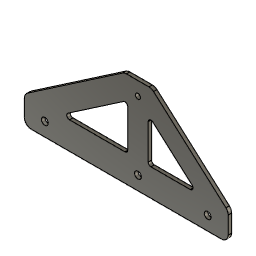
New Bell Crank with Variables v8 (Autodesk Fusion 360 design; units mm, degrees)
Autodesk Fusion 360 part; units mm, degrees
note: some values were not read from the file. Set by a fixed rule: which sketch regions a step uses.
sketch "Base Bell Crank" plane through (0, 0, 0) normal (0, 1, 0) x (1, 0, 0)
  circle A0 centre (64.9712, 0) radius 3.175
  circle A1 centre (-86.6283, 0) radius 3.175
  circle A2 centre (0, -63.5) radius 2.3813
  circle A3 centre (0, 0) radius 3.175
  line L0 (0, -63.5) -> (0, 0) construction
  line L1 (0, 0) -> (64.9712, 0) construction
  line L2 (0, 0) -> (-86.6283, 0) construction
  line L3 (-12.7, -76.2) -> (12.7, -76.2)
  line L4 (12.7, -76.2) -> (84.0212, -12.7)
  line L5 (-105.6783, 12.7) -> (-105.6783, -12.7)
  line L6 (0, -63.5) -> (0, -76.2) construction
  line L7 (64.9712, 0) -> (84.0212, 0) construction
  line L8 (84.0212, -12.7) -> (84.0212, 12.7)
  line L9 (-105.6783, 12.7) -> (84.0212, 12.7)
  line L10 (-105.6783, -12.7) -> (-12.7, -76.2)
  dimension "d12" = 4.7625
  dimension "d13" = 6.35
  dimension "d19" = 6.35
  dimension "d20" = 63.5
  dimension "d21" = 64.9712
  dimension "d22" = 86.6283
  dimension "d48" = 25.4
  dimension "d54" = 12.7
  dimension "d56" = 12.7
  dimension "d58" = 12.7
  dimension "d87" = 19.05
  dimension "d88" = 19.05
  constraint coincident A3.centre L0.end
  constraint coincident A2.centre L0.start
  constraint vertical L0
  constraint equal A0 A1
  constraint coincident A0.centre L1.end
  constraint perpendicular L0 L1
  constraint coincident A1.centre L2.end
  constraint parallel L1 L2
  constraint horizontal L3
  constraint midpoint L3 L6.end
  constraint vertical L6
  constraint horizontal L7
  constraint coincident L7.end L8
  constraint equal L5 L8
  constraint perpendicular L8 L9
  constraint horizontal L9
  constraint vertical L5
  measures "d12" diameter of A2
  measures "d13" diameter of A0
  measures "d19" diameter of A3
  measures "d20" distance of A2.centre A3.centre
  measures "d21" distance of A3.centre A0.centre
  measures "d22" distance of A1.centre A3.centre
  measures "d48" distance of L3.start L3.end
  measures "d54" vertical distance of L8.end L7.end
  measures "d56" vertical distance of L4.end L7.end
  measures "d58" distance of A2.centre L3
  measures "d87" distance of A1.centre L5
  measures "d88" distance of A0.centre L8
sketch "Sketch3" plane through (0, 0, 0) normal (0, 1, 0) x (1, 0, 0)
  line L0 (12.7, -76.2) -> (84.0212, -12.7)
  line L1 (0, -63.5) -> (0, 0)
  line L2 (0, 0) -> (64.9712, 0)
  line L3 (9.525, -53.5204) -> (9.525, -12.7)
  line L4 (9.525, -12.7) -> (55.3732, -12.7)
  line L5 (55.3732, -12.7) -> (9.525, -53.5204)
  line L6 (-9.525, -12.7) -> (-71.9004, -12.7)
  line L7 (-71.9004, -12.7) -> (-9.525, -55.2996)
  line L8 (-9.525, -55.2996) -> (-9.525, -12.7)
  line L9 (-105.6783, -12.7) -> (-12.7, -76.2)
  line L10 (-105.6783, 12.7) -> (84.0212, 12.7)
  line L11 (-9.525, -55.2996) -> (9.525, -53.5204) construction
  point P0 (0, -54.41)
  dimension "d93" = 19.05
  dimension "d96" = 19.05
  dimension "d98" = 25.4
  dimension "d103" = 19.05
  dimension "d104" = 25.4
  constraint parallel L1 L3
  constraint perpendicular L3 L4
  constraint perpendicular L1 L6
  constraint perpendicular L6 L8
  constraint parallel L7 L9
  constraint parallel L0 L5
  constraint midpoint L11 P0
  constraint coincident L1 P0
  measures "d93" distance of L7 L9
  measures "d96" distance of L3 L8
  measures "d98" distance of L6 L10
  measures "d103" distance of L0 L5
  measures "d104" distance of L4 L10
extrude "Extrude1" add sketch "Base Bell Crank" along normal blind 3.175
extrude "Extrude2" cut sketch "Sketch3" along normal up to surface (3.175 mm away)
fillet "Fillet1" radius 2.54 6 edges at (-71.9004, 1.5875, 12.7) (-9.525, 1.5875, 12.7) (-9.525, 1.5875, 55.2996) (9.525, 1.5875, 53.5204) (9.525, 1.5875, 12.7) (55.3732, 1.5875, 12.7)
fillet "Fillet2" radius 6.35 2 edges at (12.7, 1.5875, 76.2) (84.0212, 1.5875, 12.7)
fillet "Fillet2" radius 6.35 2 edges at (-105.6783, 1.5875, -12.7) (84.0212, 1.5875, -12.7)
fillet "Fillet2" radius 6.35 2 edges at (-12.7, 1.5875, 76.2) (-105.6783, 1.5875, 12.7)
equation "AngleUp = 20 deg"
equation "AngleDown = 15 deg"
equation "EyeBoltRadius = 1.4 in"
equation "EBDistCC = ( AngleUp * 3.1415 * 2 * EyeBoltRadius ) / 360 deg"
equation "EBDistCCW = ( AngleDown * 3.1415 * 2 * EyeBoltRadius ) / 360 deg"
equation "TopHoletoPivot = 2.5 in"
equation "BellCrankAngleDown = ( EBDistCCW * 360 deg ) / ( TopHoletoPivot * 3.1415 * 2 )"
equation "BellCrankAngleUp = ( EBDistCC * 360 deg ) / ( TopHoletoPivot * 3.1415 * 2 )"
equation "PullDist = 0.5 in"
equation "RightHoleDist = ( PullDist * 360 deg ) / ( 3.1415 * 2 * BellCrankAngleUp )"
equation "LeftHoleDist = ( PullDist * 360 deg ) / ( 3.1415 * 2 * BellCrankAngleDown )"
equation "d12 = TopHoleOD"
equation "d13 = CableHoleOD"
equation "TopHoleOD = ( 3 / 16 ) * 1 in"
equation "CableHoleOD = 0.25 in"
equation "StrutHoleOD = 0.25 in"
equation "d19 = StrutHoleOD"
equation "d20 = TopHoletoPivot"
equation "d21 = RightHoleDist"
equation "d22 = LeftHoleDist"
equation "d37 = ( 3 / 8 ) * 1 in"
equation "d39 = ( 3 / 8 ) * 1 in"
equation "d41 = ( 3 / 8 ) * 1 in"
equation "d83 = ( 3 / 8 ) * 1 in"
